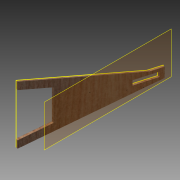
# Autodesk Inventor part: Stand
Saved by Autodesk Inventor 2017 (Build 210142000, 142)
## iProperties
Created: 2018-10-12
Part Number: Stand
Material: Wood (Birch)
Document SubType Name: Modeling
Designer: ari
Density: 0.55 g/cm^3
Appearance: Clear - Green 1
Author: ari
Autodesk Inventor part; units mm, degrees
ref_plane "XZ Plane" through (0, 0, 0) normal (0, 1, 0) x (-1, 0, 0)
ref_plane "XY Plane" through (0, 0, 0) normal (0, 0, 1) x (1, 0, 0)
sketch "Sketch1" plane through (0, 0, 0) normal (0, 0, 1) x (1, 0, 0)
  line L0 (-102.7278, -80.4997) -> (-34.2315, 155.1415)
  line L1 (-34.2315, 155.1415) -> (-39.0327, 156.5371)
  line L2 (-39.0327, 156.5371) -> (-107.529, -79.104)
  line L3 (-107.529, -79.104) -> (-102.7278, -80.4997)
  line L4 (-41.9395, 146.5371) -> (-41.9395, 156.5371) construction
  line L5 (-41.9395, 156.5371) -> (-39.0327, 156.5371) construction
  line L6 (-232.529, -80.4997) -> (-232.529, 130.1415) construction
  line L7 (-41.9395, 104.1062) -> (-418.1395, 104.1062) construction
  line L8 (-41.9395, 104.1062) -> (-41.9395, 339.3062) construction
  line L9 (-70.779, -80.4997) -> (-394.279, -80.4997) construction
  dimension "d0" = 5
  dimension "d2" = 10
  dimension "d3" = 125
  constraints: 14 end point, 2 parallel, 2 perpendicular, 1 point on line, 1 vertical
  measures "d0" distance of L2.end L0.start
  measures "d2" distance of L4.start L4.end
  measures "d3" distance from line of L6 L2.end
extrude "Extrusion1" add sketch "Sketch1" against normal blind 5
sketch "Sketch2" plane through (0, 0, 0) normal (0, 0, 1) x (1, 0, 0)
  line L0 (-102.7278, -80.4997) -> (-34.2315, 155.1415) projected
  line L1 (-34.2315, 155.1415) -> (-39.0327, 156.5371) projected
  line L2 (-39.0327, 156.5371) -> (-107.529, -79.104) projected
  line L3 (-107.529, -79.104) -> (-102.7278, -80.4997) projected
  point P0 (0, 0)
ref_plane "Work Plane1" through (-399.029, 141.4738, 12.0861) normal (0, -0.258819, -0.9659258) x (1, 0, 0)
extrude "Extrusion2" add sketch "Sketch2" along normal up to surface surface through (-399.029, 141.4738, 12.0861) normal (0, -0.258819, -0.9659258)
ref_plane "Work Plane2" through (-34.2315, 155.1415, 8.4239) normal (1, 0, 0) x (0, 1, 0)
sketch "Sketch7" plane through (0, 0, 0) normal (0, 0, 1) x (1, 0, 0)
  line L0 (-102.7278, -80.4997) -> (-34.2315, 155.1415) construction
  line L1 (-107.529, -79.104) -> (-39.0327, 156.5371) projected
  line L2 (-39.0327, 156.5371) -> (-34.2315, 155.1415)
  line L3 (-34.2315, 155.1415) -> (-47.3441, 110.0314)
  line L4 (-47.3441, 110.0314) -> (-52.1454, 111.4271)
  line L5 (-52.1454, 111.4271) -> (-39.0327, 156.5371)
  point P0 (0, 0)
  dimension "d19" = 46.9772
  constraints: 8 end point, 2 parallel, 2 perpendicular
  measures "d19" distance between parallel lines of L2 L4
extrude "Extrusion7" add sketch "Sketch7" along normal blind 15
sketch "Sketch3" plane through (-34.2315, 155.1415, 8.4239) normal (1, 0, 0) x (0, 1, 0)
  line L0 (-8.6044, -8.4239) -> (-51.0353, -8.4239) construction
  line L1 (-51.0353, -8.4239) -> (-51.0353, -0.0239) construction
  line L2 (-51.0353, -0.0239) -> (-8.6044, -0.0239) construction
  line L3 (-8.6044, -0.0239) -> (-8.6044, -8.4239) construction
  line L4 (-8.6044, -0.0239) -> (-51.0353, -8.4239) construction
  line L5 (-51.6353, 0.5761) -> (-8.0044, 0.5761)
  line L6 (-8.0044, 0.5761) -> (-8.0044, -9.0239)
  line L7 (-8.0044, -9.0239) -> (-51.6353, -9.0239)
  line L8 (-51.6353, -9.0239) -> (-51.6353, 0.5761)
  line L9 (-51.6353, 0.5761) -> (-8.0044, -9.0239) construction
  line L10 (-8.0044, 0.5761) -> (-51.6353, -9.0239) construction
  line L11 (-51.0353, -0.0239) -> (-51.0353, -8.5239) construction
  point P0 (-155.1415, -8.4239)
  point P1 (-29.8198, -4.2239)
  dimension "d10" = 0.6
  dimension "d11" = 0.6
  constraints: 22 end point, 4 parallel, 3 midpoint, 2 horizontal, 2 perpendicular
  measures "d10" distance between parallel lines of L7 L0
  measures "d11" distance between parallel lines of L6 L3
extrude "Extrusion3" cut sketch "Sketch3" along normal through all both and the other way through all
sketch "Sketch6" plane through (-102.7278, -80.4997, 71.5637) normal (0.9602541, -0.2791272, 0) x (0, 0, -1)
  line L0 (119.8334, 0) -> (76.5637, 0)
  line L1 (76.5637, 245.3946) -> (76.5637, 0) construction
  line L2 (119.8334, 0) -> (76.5637, 245.3946)
  line L3 (76.5637, 245.3946) -> (76.5637, 0)
  dimension "d16" = 10
  constraints: 6 end point, 1 collinear, 1 perpendicular
  measures "d16" angle of L2 L1
extrude "Extrusion6" add sketch "Sketch6" against normal up to surface (5 mm away)
sketch "Sketch8" plane through (-107.529, -79.104, -48.2697) normal (-0.9602541, 0.2791272, 0) x (0, 0, 1)
  line L0 (43.2697, 245.3946) -> (63.2697, 245.3946) projected
  line L1 (0, 0) -> (119.4595, 0) projected
  line L2 (63.2697, 218.3829) -> (119.4595, 0) projected
  line L3 (63.2697, 245.3946) -> (63.2697, 218.3829) projected
  line L4 (57.2697, 235.6055) -> (57.2697, 190.1687) projected
  line L5 (57.2697, 190.1687) -> (47.6697, 190.1687) projected
  line L6 (47.6697, 190.1687) -> (47.6697, 235.6055) projected
  line L7 (47.6697, 235.6055) -> (57.2697, 235.6055) projected
  line L8 (0, 0) -> (43.2697, 245.3946) projected
  point P0 (48.2697, 105.9743)
fillet "Fillet1" radius 2 2 edges at (-36.6321, 155.8393, -5) (-36.6321, 155.8393, 15)
fillet "Fillet1" radius 20 1 edges at (-43.969, 130.5991, 15)
sketch "Sketch9" plane through (-102.7278, -80.4997, 71.5637) normal (0.9602541, -0.2791272, 0) x (0, 0, -1)
  line L0 (0, 0) -> (55.8822, 217.1877) construction
  line L1 (76.8551, 243.7419) -> (119.8334, 0) construction
  line L2 (15, 0) -> (30.438, 60)
  line L3 (30.438, 60) -> (94.2538, 60)
  line L4 (94.2538, 60) -> (104.8334, 0)
  line L5 (15, 0) -> (104.8334, 0)
  line L6 (0, 0) -> (15, 0) construction
  line L7 (119.8334, 0) -> (76.8551, 243.7419) construction
  line L8 (104.8334, 0) -> (119.8334, 0) construction
  point P0 (71.5637, 105.9743)
  dimension "d24" = 15
  dimension "d25" = 60
  constraints: 12 end point, 2 collinear, 2 parallel, 1 horizontal
  measures "d24" distance of L0.start L2.start
  measures "d25" distance between parallel lines of L5 L3
extrude "Extrusion8" cut sketch "Sketch9" against normal through all
ref_plane "Work Plane5" through (-49.2408, 103.5062, 4.2) normal (0, 0, -1) x (-1, 0, 0)
sketch "Sketch10" plane through (-49.2408, 103.5062, 4.2) normal (0, 0, -1) x (-1, 0, 0)
  line L0 (5.2337, -27.2953) -> (13.8107, -29.5988) construction
  line L1 (6.5305, -22.4664) -> (5.2337, -27.2953) construction
  line L2 (15.1076, -24.7699) -> (6.5305, -22.4664) construction
  line L3 (13.8107, -29.5988) -> (15.1076, -24.7699) construction
  line L4 (-14.5481, 50.0483) -> (-9.7468, 51.4439) construction
  line L5 (-14.5481, 50.0483) -> (53.4869, -184.0059) construction
  line L6 (53.4869, -184.0059) -> (58.2882, -182.6103) construction
  line L7 (58.2882, -182.6103) -> (-9.7468, 51.4439) construction
  line L8 (53.4869, -184.0059) -> (-7.1361, 24.5495) construction
  line L9 (6.5305, -22.4664) -> (11.3318, -21.0707)
  line L10 (11.3318, -21.0707) -> (13.8107, -29.5988)
  line L11 (13.8107, -29.5988) -> (9.0095, -30.9944)
  line L12 (9.0095, -30.9944) -> (6.5305, -22.4664)
  line L13 (58.2882, -182.6103) -> (-9.7468, 51.4439) construction
  point P0 (-49.2408, -103.5062)
  constraints: 28 end point, 2 parallel, 2 perpendicular, 2 point on line, 1 coincident
extrude "Extrusion9" cut sketch "Sketch10" along normal through all
sketch "Sketch12" plane through (-49.2408, 103.5062, 4.2) normal (0, 0, -1) x (-1, 0, 0)
  line L0 (36.7393, -126.3907) -> (41.5406, -124.995) construction
  line L1 (36.7393, -126.3907) -> (41.5406, -124.995) construction
  line L2 (13.8107, -29.5988) -> (9.0095, -30.9944) construction
  line L3 (9.0095, -30.9944) -> (53.4869, -184.0059) construction
  line L4 (53.4869, -184.0059) -> (58.2882, -182.6103) construction
  line L5 (58.2882, -182.6103) -> (13.8107, -29.5988) construction
  line L6 (33.3898, -114.8676) -> (31.9941, -110.0663)
  line L7 (31.9941, -110.0663) -> (36.7954, -108.6707)
  line L8 (36.7954, -108.6707) -> (38.191, -113.472)
  line L9 (38.191, -113.472) -> (33.3898, -114.8676)
  point P0 (-49.2408, -103.5062)
  dimension "d32" = 12
  dimension "d33" = 5
  constraints: 8 end point, 3 point on line, 2 parallel, 1 perpendicular
  measures "d32" distance between parallel lines of L0 L9
  measures "d33" distance between parallel lines of L9 L7
extrude "Extrusion10" cut sketch "Sketch12" along normal through all
body "Solid1"
